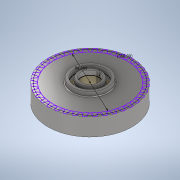
# Autodesk Inventor part: Practica 18
Saved by Autodesk Inventor 2020 (Build 240168000, 168)
## iProperties
Created: 2020-03-03
Part Number: Practica 18
Material: Acero inoxidable
Document SubType Name: Chapa
Designer: Luis Gallardo
Density: 8 g/cm^3
Sheet Metal Rule: Por defecto_mm
Appearance: Galvanizado
Author: Luis Gallardo
Autodesk Inventor part; units mm, degrees
ref_plane "YZ Plane" through (0, 0, 0) normal (1, 0, 0) x (0, 1, 0)
ref_plane "XZ Plane" through (0, 0, 0) normal (0, 1, 0) x (-1, 0, 0)
ref_plane "XY Plane" through (0, 0, 0) normal (0, 0, 1) x (1, 0, 0)
sketch "Boceto1" plane through (0, 0, 0) normal (0, 1, 0) x (-1, 0, 0)
  circle A0 centre (0, 0) radius 47.5
  circle A1 centre (0, 0) radius 10
  dimension "d0" = 95
  dimension "d1" = 20
  constraints: 2 centre point, 2 coincident
  measures "d0" diameter of A0
  measures "d1" diameter of A1
extrude "Extrusión1" add sketch "Boceto1" along normal blind 20
sketch "Boceto3" plane through (0, 20, 0) normal (0, 1, 0) x (1, 0, 0)
  circle A0 centre (0, 0) radius 10
  circle A1 centre (0, 0) radius 12.5
  circle A2 centre (0, 0) radius 17
  circle A3 centre (0, 0) radius 20
  dimension "d18" = 20
  dimension "d19" = 25
  dimension "d20" = 34
  dimension "d21" = 40
  constraints: 4 centre point, 4 coincident
  measures "d18" diameter of A0
  measures "d19" diameter of A1
  measures "d20" diameter of A2
  measures "d21" diameter of A3
extrude "Extrusión3" add sketch "Boceto3" along normal blind 5 contours A1
extrude "Extrusión4" add sketch "Boceto3" along normal blind 5 contours A3
fillet "Empalme1" radius 1 2 edges at (-20, 20, 0) (-12.5, 20, 0)
sketch "Boceto4" plane through (0, 25, 0) normal (0, 1, 0) x (1, 0, 0)
  circle A0 centre (0, 0) radius 12.5 projected
  circle A1 centre (0, 0) radius 10 projected
  line L0 (-2.0947, 12.3232) -> (1.8315, 12.3232)
  line L1 (1.8315, 12.3232) -> (1.8315, 9.8308)
  line L2 (1.8315, 9.8308) -> (-2.0947, 9.8308)
  line L3 (-2.0947, 9.8308) -> (-2.0947, 12.3232)
  point P0 (-1.8315, 9.8308)
  constraints: 8 end point, 2 parallel, 1 horizontal, 1 perpendicular, 4 other
extrude "Extrusión5" cut sketch "Boceto4" against normal through all contours L0 L1 A1 L2 L3
ref_plane "Plano de trabajo1" through (0, 20, 0) normal (0, 1, 0) x (1, 0, 0)
sketch "Boceto5" plane through (0, 20, 0) normal (0, 1, 0) x (1, 0, 0)
  arc A0 (-5.7983, 45.129) -> (-6.6944, 47.0259) centre (-9.668, 44.461) ccw
  arc A1 (-9.4598, 46.5485) -> (-9.596, 44.1298) centre (-5.7983, 45.129) ccw
  arc A2 (-5.7983, 45.129) -> (-3.5136, 41.8874) centre (-1.8853, 45.4609) ccw
  arc A3 (-10.7336, 40.641) -> (-9.596, 44.1298) centre (-13.4658, 43.4617) ccw
  arc A4 (-6.6944, 47.0259) -> (-9.4598, 46.5485) centre (0, 0) ccw
  circle A5 centre (0, 0) radius 42.0345
  arc A6 (-17.3991, 44.1987) -> (-17.1133, 41.793) centre (-13.5468, 43.4366) ccw
  arc A7 (-17.6278, 38.1597) -> (-17.1133, 41.793) centre (-20.8083, 40.4631) ccw
  arc A8 (-14.7587, 45.149) -> (-17.3991, 44.1987) centre (0, 0) ccw
  arc A9 (-13.5468, 43.4366) -> (-14.7587, 45.149) centre (-17.2417, 42.1067) ccw
  arc A10 (-13.5468, 43.4366) -> (-10.7339, 40.6409) centre (-9.7509, 44.4429) ccw
  circle A11 centre (0, 0) radius 42.0345
  arc A12 (-24.8098, 40.5059) -> (-24.1106, 38.1864) centre (-20.8836, 40.4243) ccw
  arc A13 (-23.9864, 34.5189) -> (-24.1106, 38.1864) centre (-27.5185, 36.2351) ccw
  arc A14 (-22.3745, 41.9003) -> (-24.8098, 40.5059) centre (0, 0) ccw
  arc A15 (-20.8836, 40.4243) -> (-22.3745, 41.9003) centre (-24.2915, 38.473) ccw
  arc A16 (-20.8836, 40.4243) -> (-17.628, 38.1596) centre (-17.3202, 42.0745) ccw
  circle A17 centre (0, 0) radius 42.0345
  arc A18 (-31.4666, 35.5823) -> (-30.3753, 33.4195) centre (-27.586, 36.1838) ccw
  arc A19 (-29.6161, 29.8293) -> (-30.3753, 33.4195) centre (-33.3926, 30.9061) ccw
  arc A20 (-29.3105, 37.3784) -> (-31.4666, 35.5823) centre (0, 0) ccw
  arc A21 (-27.586, 36.1838) -> (-29.3105, 37.3784) centre (-30.6033, 33.6703) ccw
  arc A22 (-27.586, 36.1838) -> (-23.9866, 34.5188) centre (-24.3632, 38.4277) ccw
  circle A23 centre (0, 0) radius 42.0345
  arc A24 (-37.1674, 29.5776) -> (-35.7171, 27.6372) centre (-33.4501, 30.8438) ccw
  arc A25 (-34.346, 24.2333) -> (-35.7171, 27.6372) centre (-38.2521, 24.638) ccw
  arc A26 (-35.3559, 31.7209) -> (-37.1674, 29.5776) centre (0, 0) ccw
  arc A27 (-33.4501, 30.8438) -> (-35.3559, 31.7209) centre (-35.9851, 27.8446) ccw
  arc A28 (-33.4501, 30.8438) -> (-29.6163, 29.8291) centre (-30.666, 33.6132) ccw
  circle A29 centre (0, 0) radius 42.0345
  arc A30 (-41.7388, 22.6742) -> (-39.9736, 21.0151) centre (-38.2979, 24.5666) ccw
  arc A31 (-38.0322, 17.9011) -> (-39.9736, 21.0151) centre (-41.9493, 17.6213) ccw
  arc A32 (-40.327, 25.0995) -> (-41.7388, 22.6742) centre (0, 0) ccw
  arc A33 (-38.2979, 24.5666) -> (-40.327, 25.0995) centre (-40.2736, 21.1728) ccw
  arc A34 (-38.2979, 24.5666) -> (-34.3461, 24.2331) centre (-36.037, 27.7775) ccw
  circle A35 centre (0, 0) radius 42.0345
  arc A36 (-45.0421, 15.0819) -> (-43.0155, 13.7545) centre (-41.982, 17.5431) ccw
  arc A37 (-40.5629, 11.0249) -> (-43.0155, 13.7545) centre (-44.3719, 10.0692) ccw
  arc A38 (-44.0728, 17.7154) -> (-45.0421, 15.0819) centre (0, 0) ccw
  arc A39 (-41.982, 17.5431) -> (-44.0728, 17.7154) centre (-43.3384, 13.8577) ccw
  arc A40 (-41.982, 17.5431) -> (-38.0323, 17.9008) centre (-40.313, 21.0977) ccw
  circle A41 centre (0, 0) radius 42.0345
  arc A42 (-46.9767, 7.0313) -> (-44.7505, 6.076) centre (-44.3906, 9.9864) ccw
  arc A43 (-41.8611, 3.8137) -> (-44.7505, 6.076) centre (-45.4462, 2.2111) ccw
  arc A44 (-46.4795, 9.7931) -> (-46.9767, 7.0313) centre (0, 0) ccw
  arc A45 (-44.3906, 9.9864) -> (-46.4795, 9.7931) centre (-45.0863, 6.1216) ccw
  arc A46 (-44.3906, 9.9864) -> (-40.563, 11.0246) centre (-43.3641, 13.7769) ccw
  circle A47 centre (0, 0) radius 42.0345
  arc A48 (-47.484, -1.233) -> (-45.1257, -1.7872) centre (-45.4503, 2.1264) ccw
  arc A49 (-41.8874, -3.5133) -> (-45.1257, -1.7872) centre (-45.1398, -5.7142) ccw
  arc A50 (-47.4739, 1.5733) -> (-47.484, -1.233) centre (0, 0) ccw
  arc A51 (-45.4503, 2.1264) -> (-47.4739, 1.5733) centre (-45.4644, -1.8006) ccw
  arc A52 (-45.4503, 2.1264) -> (-41.8612, 3.8135) centre (-45.0977, 6.0375) ccw
  circle A53 centre (0, 0) radius 42.0345
  arc A54 (-46.5485, -9.4598) -> (-44.1298, -9.596) centre (-45.129, -5.7983) ccw
  arc A55 (-40.641, -10.7336) -> (-44.1298, -9.596) centre (-43.4617, -13.4658) ccw
  arc A56 (-47.0259, -6.6944) -> (-46.5485, -9.4598) centre (0, 0) ccw
  arc A57 (-45.129, -5.7983) -> (-47.0259, -6.6944) centre (-44.461, -9.668) ccw
  arc A58 (-45.129, -5.7983) -> (-41.8874, -3.5136) centre (-45.4609, -1.8853) ccw
  circle A59 centre (0, 0) radius 42.0345
  arc A60 (-44.1987, -17.3991) -> (-41.793, -17.1133) centre (-43.4366, -13.5468) ccw
  arc A61 (-38.1597, -17.6278) -> (-41.793, -17.1133) centre (-40.4631, -20.8083) ccw
  arc A62 (-45.149, -14.7587) -> (-44.1987, -17.3991) centre (0, 0) ccw
  arc A63 (-43.4366, -13.5468) -> (-45.149, -14.7587) centre (-42.1067, -17.2417) ccw
  arc A64 (-43.4366, -13.5468) -> (-40.6409, -10.7339) centre (-44.4429, -9.7509) ccw
  circle A65 centre (0, 0) radius 42.0345
  arc A66 (-40.5059, -24.8098) -> (-38.1864, -24.1106) centre (-40.4243, -20.8836) ccw
  arc A67 (-34.5189, -23.9864) -> (-38.1864, -24.1106) centre (-36.2351, -27.5185) ccw
  arc A68 (-41.9003, -22.3745) -> (-40.5059, -24.8098) centre (0, 0) ccw
  arc A69 (-40.4243, -20.8836) -> (-41.9003, -22.3745) centre (-38.473, -24.2915) ccw
  arc A70 (-40.4243, -20.8836) -> (-38.1596, -17.628) centre (-42.0745, -17.3202) ccw
  circle A71 centre (0, 0) radius 42.0345
  arc A72 (-35.5823, -31.4666) -> (-33.4195, -30.3753) centre (-36.1838, -27.586) ccw
  arc A73 (-29.8293, -29.6161) -> (-33.4195, -30.3753) centre (-30.9061, -33.3926) ccw
  arc A74 (-37.3784, -29.3105) -> (-35.5823, -31.4666) centre (0, 0) ccw
  arc A75 (-36.1838, -27.586) -> (-37.3784, -29.3105) centre (-33.6703, -30.6033) ccw
  arc A76 (-36.1838, -27.586) -> (-34.5188, -23.9866) centre (-38.4277, -24.3632) ccw
  circle A77 centre (0, 0) radius 42.0345
  arc A78 (-29.5776, -37.1674) -> (-27.6372, -35.7171) centre (-30.8438, -33.4501) ccw
  arc A79 (-24.2333, -34.346) -> (-27.6372, -35.7171) centre (-24.638, -38.2521) ccw
  arc A80 (-31.7209, -35.3559) -> (-29.5776, -37.1674) centre (0, 0) ccw
  arc A81 (-30.8438, -33.4501) -> (-31.7209, -35.3559) centre (-27.8446, -35.9851) ccw
  arc A82 (-30.8438, -33.4501) -> (-29.8291, -29.6163) centre (-33.6132, -30.666) ccw
  circle A83 centre (0, 0) radius 42.0345
  arc A84 (-22.6742, -41.7388) -> (-21.0151, -39.9736) centre (-24.5666, -38.2979) ccw
  arc A85 (-17.9011, -38.0322) -> (-21.0151, -39.9736) centre (-17.6213, -41.9493) ccw
  arc A86 (-25.0995, -40.327) -> (-22.6742, -41.7388) centre (0, 0) ccw
  arc A87 (-24.5666, -38.2979) -> (-25.0995, -40.327) centre (-21.1728, -40.2736) ccw
  arc A88 (-24.5666, -38.2979) -> (-24.2331, -34.3461) centre (-27.7775, -36.037) ccw
  circle A89 centre (0, 0) radius 42.0345
  arc A90 (-15.0819, -45.0421) -> (-13.7545, -43.0155) centre (-17.5431, -41.982) ccw
  arc A91 (-11.0249, -40.5629) -> (-13.7545, -43.0155) centre (-10.0692, -44.3719) ccw
  arc A92 (-17.7154, -44.0728) -> (-15.0819, -45.0421) centre (0, 0) ccw
  arc A93 (-17.5431, -41.982) -> (-17.7154, -44.0728) centre (-13.8577, -43.3384) ccw
  arc A94 (-17.5431, -41.982) -> (-17.9008, -38.0323) centre (-21.0977, -40.313) ccw
  circle A95 centre (0, 0) radius 42.0345
  arc A96 (-7.0313, -46.9767) -> (-6.076, -44.7505) centre (-9.9864, -44.3906) ccw
  arc A97 (-3.8137, -41.8611) -> (-6.076, -44.7505) centre (-2.2111, -45.4462) ccw
  arc A98 (-9.7931, -46.4795) -> (-7.0313, -46.9767) centre (0, 0) ccw
  arc A99 (-9.9864, -44.3906) -> (-9.7931, -46.4795) centre (-6.1216, -45.0863) ccw
  arc A100 (-9.9864, -44.3906) -> (-11.0246, -40.563) centre (-13.7769, -43.3641) ccw
  circle A101 centre (0, 0) radius 42.0345
  arc A102 (1.233, -47.484) -> (1.7872, -45.1257) centre (-2.1264, -45.4503) ccw
  arc A103 (3.5133, -41.8874) -> (1.7872, -45.1257) centre (5.7142, -45.1398) ccw
  arc A104 (-1.5733, -47.4739) -> (1.233, -47.484) centre (0, 0) ccw
  arc A105 (-2.1264, -45.4503) -> (-1.5733, -47.4739) centre (1.8006, -45.4644) ccw
  arc A106 (-2.1264, -45.4503) -> (-3.8135, -41.8612) centre (-6.0375, -45.0977) ccw
  circle A107 centre (0, 0) radius 42.0345
  arc A108 (9.4598, -46.5485) -> (9.596, -44.1298) centre (5.7983, -45.129) ccw
  arc A109 (10.7336, -40.641) -> (9.596, -44.1298) centre (13.4658, -43.4617) ccw
  arc A110 (6.6944, -47.0259) -> (9.4598, -46.5485) centre (0, 0) ccw
  arc A111 (5.7983, -45.129) -> (6.6944, -47.0259) centre (9.668, -44.461) ccw
  arc A112 (5.7983, -45.129) -> (3.5136, -41.8874) centre (1.8853, -45.4609) ccw
  circle A113 centre (0, 0) radius 42.0345
  arc A114 (17.3991, -44.1987) -> (17.1133, -41.793) centre (13.5468, -43.4366) ccw
  arc A115 (17.6278, -38.1597) -> (17.1133, -41.793) centre (20.8083, -40.4631) ccw
  arc A116 (14.7587, -45.149) -> (17.3991, -44.1987) centre (0, 0) ccw
  arc A117 (13.5468, -43.4366) -> (14.7587, -45.149) centre (17.2417, -42.1067) ccw
  arc A118 (13.5468, -43.4366) -> (10.7339, -40.6409) centre (9.7509, -44.4429) ccw
  circle A119 centre (0, 0) radius 42.0345
  arc A120 (24.8098, -40.5059) -> (24.1106, -38.1864) centre (20.8836, -40.4243) ccw
  arc A121 (23.9864, -34.5189) -> (24.1106, -38.1864) centre (27.5185, -36.2351) ccw
  arc A122 (22.3745, -41.9003) -> (24.8098, -40.5059) centre (0, 0) ccw
  arc A123 (20.8836, -40.4243) -> (22.3745, -41.9003) centre (24.2915, -38.473) ccw
  arc A124 (20.8836, -40.4243) -> (17.628, -38.1596) centre (17.3202, -42.0745) ccw
  circle A125 centre (0, 0) radius 42.0345
  arc A126 (31.4666, -35.5823) -> (30.3753, -33.4195) centre (27.586, -36.1838) ccw
  arc A127 (29.6161, -29.8293) -> (30.3753, -33.4195) centre (33.3926, -30.9061) ccw
  arc A128 (29.3105, -37.3784) -> (31.4666, -35.5823) centre (0, 0) ccw
  arc A129 (27.586, -36.1838) -> (29.3105, -37.3784) centre (30.6033, -33.6703) ccw
  arc A130 (27.586, -36.1838) -> (23.9866, -34.5188) centre (24.3632, -38.4277) ccw
  circle A131 centre (0, 0) radius 42.0345
  arc A132 (37.1674, -29.5776) -> (35.7171, -27.6372) centre (33.4501, -30.8438) ccw
  arc A133 (34.346, -24.2333) -> (35.7171, -27.6372) centre (38.2521, -24.638) ccw
  arc A134 (35.3559, -31.7209) -> (37.1674, -29.5776) centre (0, 0) ccw
  arc A135 (33.4501, -30.8438) -> (35.3559, -31.7209) centre (35.9851, -27.8446) ccw
  arc A136 (33.4501, -30.8438) -> (29.6163, -29.8291) centre (30.666, -33.6132) ccw
  circle A137 centre (0, 0) radius 42.0345
  arc A138 (41.7388, -22.6742) -> (39.9736, -21.0151) centre (38.2979, -24.5666) ccw
  arc A139 (38.0322, -17.9011) -> (39.9736, -21.0151) centre (41.9493, -17.6213) ccw
  arc A140 (40.327, -25.0995) -> (41.7388, -22.6742) centre (0, 0) ccw
  arc A141 (38.2979, -24.5666) -> (40.327, -25.0995) centre (40.2736, -21.1728) ccw
  arc A142 (38.2979, -24.5666) -> (34.3461, -24.2331) centre (36.037, -27.7775) ccw
  circle A143 centre (0, 0) radius 42.0345
  arc A144 (45.0421, -15.0819) -> (43.0155, -13.7545) centre (41.982, -17.5431) ccw
  arc A145 (40.5629, -11.0249) -> (43.0155, -13.7545) centre (44.3719, -10.0692) ccw
  arc A146 (44.0728, -17.7154) -> (45.0421, -15.0819) centre (0, 0) ccw
  arc A147 (41.982, -17.5431) -> (44.0728, -17.7154) centre (43.3384, -13.8577) ccw
  arc A148 (41.982, -17.5431) -> (38.0323, -17.9008) centre (40.313, -21.0977) ccw
  circle A149 centre (0, 0) radius 42.0345
  arc A150 (46.9767, -7.0313) -> (44.7505, -6.076) centre (44.3906, -9.9864) ccw
  arc A151 (41.8611, -3.8137) -> (44.7505, -6.076) centre (45.4462, -2.2111) ccw
  arc A152 (46.4795, -9.7931) -> (46.9767, -7.0313) centre (0, 0) ccw
  arc A153 (44.3906, -9.9864) -> (46.4795, -9.7931) centre (45.0863, -6.1216) ccw
  arc A154 (44.3906, -9.9864) -> (40.563, -11.0246) centre (43.3641, -13.7769) ccw
  circle A155 centre (0, 0) radius 42.0345
  arc A156 (47.484, 1.233) -> (45.1257, 1.7872) centre (45.4503, -2.1264) ccw
  arc A157 (41.8874, 3.5133) -> (45.1257, 1.7872) centre (45.1398, 5.7142) ccw
  arc A158 (47.4739, -1.5733) -> (47.484, 1.233) centre (0, 0) ccw
  arc A159 (45.4503, -2.1264) -> (47.4739, -1.5733) centre (45.4644, 1.8006) ccw
  arc A160 (45.4503, -2.1264) -> (41.8612, -3.8135) centre (45.0977, -6.0375) ccw
  circle A161 centre (0, 0) radius 42.0345
  arc A162 (46.5485, 9.4598) -> (44.1298, 9.596) centre (45.129, 5.7983) ccw
  arc A163 (40.641, 10.7336) -> (44.1298, 9.596) centre (43.4617, 13.4658) ccw
  arc A164 (47.0259, 6.6944) -> (46.5485, 9.4598) centre (0, 0) ccw
  arc A165 (45.129, 5.7983) -> (47.0259, 6.6944) centre (44.461, 9.668) ccw
  arc A166 (45.129, 5.7983) -> (41.8874, 3.5136) centre (45.4609, 1.8853) ccw
  circle A167 centre (0, 0) radius 42.0345
  arc A168 (44.1987, 17.3991) -> (41.793, 17.1133) centre (43.4366, 13.5468) ccw
  arc A169 (38.1597, 17.6278) -> (41.793, 17.1133) centre (40.4631, 20.8083) ccw
  arc A170 (45.149, 14.7587) -> (44.1987, 17.3991) centre (0, 0) ccw
  arc A171 (43.4366, 13.5468) -> (45.149, 14.7587) centre (42.1067, 17.2417) ccw
  arc A172 (43.4366, 13.5468) -> (40.6409, 10.7339) centre (44.4429, 9.7509) ccw
  circle A173 centre (0, 0) radius 42.0345
  arc A174 (40.5059, 24.8098) -> (38.1864, 24.1106) centre (40.4243, 20.8836) ccw
  arc A175 (34.5189, 23.9864) -> (38.1864, 24.1106) centre (36.2351, 27.5185) ccw
  arc A176 (41.9003, 22.3745) -> (40.5059, 24.8098) centre (0, 0) ccw
  arc A177 (40.4243, 20.8836) -> (41.9003, 22.3745) centre (38.473, 24.2915) ccw
  arc A178 (40.4243, 20.8836) -> (38.1596, 17.628) centre (42.0745, 17.3202) ccw
  circle A179 centre (0, 0) radius 42.0345
  arc A180 (35.5823, 31.4666) -> (33.4195, 30.3753) centre (36.1838, 27.586) ccw
  arc A181 (29.8293, 29.6161) -> (33.4195, 30.3753) centre (30.9061, 33.3926) ccw
  arc A182 (37.3784, 29.3105) -> (35.5823, 31.4666) centre (0, 0) ccw
  arc A183 (36.1838, 27.586) -> (37.3784, 29.3105) centre (33.6703, 30.6033) ccw
  arc A184 (36.1838, 27.586) -> (34.5188, 23.9866) centre (38.4277, 24.3632) ccw
  circle A185 centre (0, 0) radius 42.0345
  arc A186 (29.5776, 37.1674) -> (27.6372, 35.7171) centre (30.8438, 33.4501) ccw
  arc A187 (24.2333, 34.346) -> (27.6372, 35.7171) centre (24.638, 38.2521) ccw
  arc A188 (31.7209, 35.3559) -> (29.5776, 37.1674) centre (0, 0) ccw
  arc A189 (30.8438, 33.4501) -> (31.7209, 35.3559) centre (27.8446, 35.9851) ccw
  arc A190 (30.8438, 33.4501) -> (29.8291, 29.6163) centre (33.6132, 30.666) ccw
  circle A191 centre (0, 0) radius 42.0345
  arc A192 (22.6742, 41.7388) -> (21.0151, 39.9736) centre (24.5666, 38.2979) ccw
  arc A193 (17.9011, 38.0322) -> (21.0151, 39.9736) centre (17.6213, 41.9493) ccw
  arc A194 (25.0995, 40.327) -> (22.6742, 41.7388) centre (0, 0) ccw
  arc A195 (24.5666, 38.2979) -> (25.0995, 40.327) centre (21.1728, 40.2736) ccw
  arc A196 (24.5666, 38.2979) -> (24.2331, 34.3461) centre (27.7775, 36.037) ccw
  circle A197 centre (0, 0) radius 42.0345
  arc A198 (15.0819, 45.0421) -> (13.7545, 43.0155) centre (17.5431, 41.982) ccw
  arc A199 (11.0249, 40.5629) -> (13.7545, 43.0155) centre (10.0692, 44.3719) ccw
  arc A200 (17.7154, 44.0728) -> (15.0819, 45.0421) centre (0, 0) ccw
  arc A201 (17.5431, 41.982) -> (17.7154, 44.0728) centre (13.8577, 43.3384) ccw
  arc A202 (17.5431, 41.982) -> (17.9008, 38.0323) centre (21.0977, 40.313) ccw
  circle A203 centre (0, 0) radius 42.0345
  arc A204 (7.0313, 46.9767) -> (6.076, 44.7505) centre (9.9864, 44.3906) ccw
  arc A205 (3.8137, 41.8611) -> (6.076, 44.7505) centre (2.2111, 45.4462) ccw
  arc A206 (9.7931, 46.4795) -> (7.0313, 46.9767) centre (0, 0) ccw
  arc A207 (9.9864, 44.3906) -> (9.7931, 46.4795) centre (6.1216, 45.0863) ccw
  arc A208 (9.9864, 44.3906) -> (11.0246, 40.563) centre (13.7769, 43.3641) ccw
  circle A209 centre (0, 0) radius 42.0345
  arc A210 (-1.233, 47.484) -> (-1.7872, 45.1257) centre (2.1264, 45.4503) ccw
  arc A211 (-3.5133, 41.8874) -> (-1.7872, 45.1257) centre (-5.7142, 45.1398) ccw
  arc A212 (1.5733, 47.4739) -> (-1.233, 47.484) centre (0, 0) ccw
  arc A213 (2.1264, 45.4503) -> (1.5733, 47.4739) centre (-1.8006, 45.4644) ccw
  arc A214 (2.1264, 45.4503) -> (3.8135, 41.8612) centre (6.0375, 45.0977) ccw
  circle A215 centre (0, 0) radius 42.0345
  point P0 (-9.7125, 44.6168)
  dimension "d47" = 84.069
  dimension "d50" = 360
  constraints: 432 point on circle, 216 centre point, 38 coincident, 611 other
  measures "d47" diameter of A5
equation "\"Radio_pliegue\" = Grosor"
equation "\"Anchura_desahogo_plegado\" = Grosor"
equation "\"Profundidad_desahogo_plegado\" = 0.5 * Grosor"
equation "\"Tamaño_destalonado\" = 4 * Grosor"
equation "\"Remanente_mínimo\" = 2 * Grosor"
equation "\"Radiodetransición\" = Radio_pliegue"
equation "\"Tamaño_de_radio_de_Jacobi\" = Radio_pliegue"
equation "\"TamañoSeparación\" = Grosor"
equation "\"Grosor\" = 0.5"
